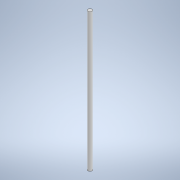
# Autodesk Inventor part: Shaft (Connecting First Link to Second Link) V5
Saved by Autodesk Inventor 2022 (Build 260153000, 153)
## iProperties
Created: 2021-10-31
Part Number: Shaft (Connecting First Link to Second Link) V5
Material: Generic
Document SubType Name: Modeling
Designer: shubh
Density: 1 g/cm^3
Appearance: Default
Mass: 458.74 g
Surface Area: 453.35 cm^2
Volume: 458.74 cm^3
Author: shubh
Autodesk Inventor part; units mm, degrees
ref_plane "YZ Plane" through (0, 0, 0) normal (1, 0, 0) x (0, 1, 0)
ref_plane "XZ Plane" through (0, 0, 0) normal (0, 1, 0) x (-1, 0, 0)
ref_plane "XY Plane" through (0, 0, 0) normal (0, 0, 1) x (1, 0, 0)
sketch "Sketch1" plane through (0, 0, 0) normal (0, 1, 0) x (-1, 0, 0)
  circle A0 centre (0, 0) radius 4
  dimension "shaft_diameter" = 8
  constraints: 1 centre point, 1 coincident
  measures "shaft_diameter" diameter of A0
extrude "Extrusion1" add sketch "Sketch1" along normal blind 279.4
body "Solid1"
